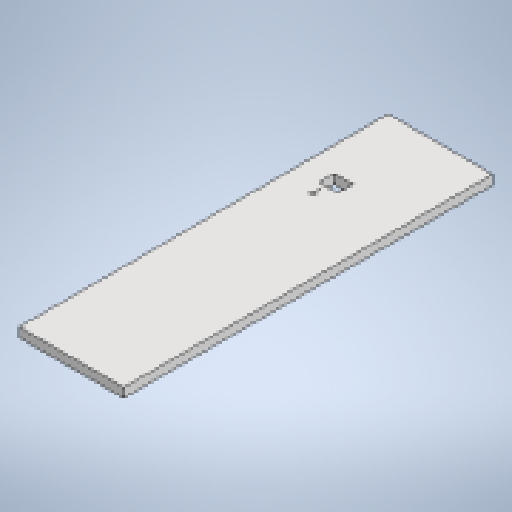
# Autodesk Inventor part: GnG foundation
Saved by Autodesk Inventor 2025 (Build 290162010, 162A)
## iProperties
Created: 2025-11-07
Part Number: GnG foundation
Material: Generic
Document SubType Name: Modeling
Designer: admin
Density: 1 g/cm^3
Appearance: Default
Author: admin
Autodesk Inventor part; units mm, degrees
ref_plane "YZ Plane" through (0, 0, 0) normal (1, 0, 0) x (0, 1, 0)
ref_plane "XZ Plane" through (0, 0, 0) normal (0, 1, 0) x (-1, 0, 0)
ref_plane "XY Plane" through (0, 0, 0) normal (0, 0, 1) x (1, 0, 0)
sketch "Sketch1" plane through (0, 0, 0) normal (0, 0, 1) x (1, 0, 0)
  line L0 (-1700, 6000) -> (1700, 6000)
  line L1 (1700, 6000) -> (1700, -6000)
  line L2 (1700, -6000) -> (-1700, -6000)
  line L3 (-1700, -6000) -> (-1700, 6000)
  line L4 (-1700, 6000) -> (1700, -6000) construction
  line L5 (1700, 6000) -> (-1700, -6000) construction
  line L6 (-900, 3450) -> (-300, 3450)
  line L7 (-300, 3450) -> (-300, 2950)
  line L8 (-300, 2950) -> (-900, 2950)
  line L9 (-900, 2950) -> (-900, 3450)
  line L10 (-900, 3450) -> (-300, 2950) construction
  line L11 (-300, 3450) -> (-900, 2950) construction
  circle A0 centre (-700, 1950) radius 84
  circle A1 centre (-700, 2150) radius 31.5
  point P0 (0, 0)
  point P1 (-600, 3200)
  dimension "d0" = 3400
  dimension "d1" = 12000
  dimension "d2" = 600
  dimension "d3" = 500
  dimension "d4" = 168
  dimension "d5" = 63
  dimension "d6" = 1000
  dimension "d7" = 800
  dimension "d10" = 2550
  dimension "d11" = 3850
  dimension "d12" = 200
  constraints: 24 end point, 4 midpoint, 4 parallel, 2 centre point, 2 horizontal, 2 perpendicular, 1 vertical alignment
  measures "d0" distance of L1.end L2.end
  measures "d1" distance of L0.end L1.end
  measures "d2" distance of L7.end L8.end
  measures "d3" distance of L6.end L7.end
  measures "d4" diameter of A0
  measures "d5" diameter of A1
  measures "d6" distance from line of A1.centre L3
  measures "d7" distance between parallel lines of L3 L9
  measures "d10" distance between parallel lines of L6 L0
  measures "d11" distance from line of A1.centre L0
  measures "d12" distance of A0.centre A1.centre
extrude "Extrusion1" add sketch "Sketch1" against normal blind 300
body "Solid1"
